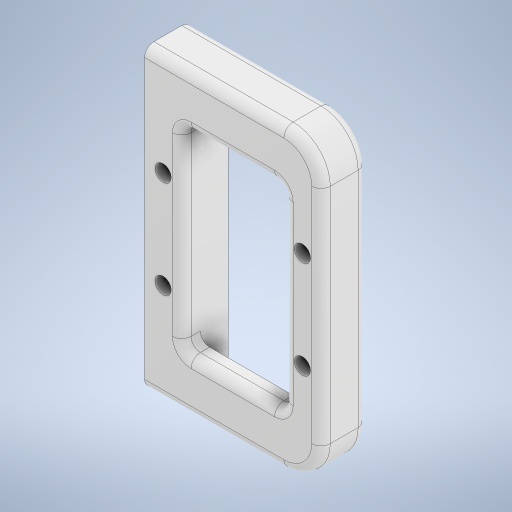
# Autodesk Inventor part: CoxaLeft
Saved by Autodesk Inventor 2024 (Build 280153000, 153)
## iProperties
Created: 2026-01-13
Part Number: CoxaLeft
Material: Generic
Document SubType Name: Modeling
Designer: Liam
Density: 1 g/cm^3
Appearance: Default
Author: Liam
Autodesk Inventor part; units mm, degrees
ref_plane "YZ Plane" through (0, 0, 0) normal (1, 0, 0) x (0, 1, 0)
ref_plane "XZ Plane" through (0, 0, 0) normal (0, 1, 0) x (-1, 0, 0)
ref_plane "XY Plane" through (0, 0, 0) normal (0, 0, 1) x (1, 0, 0)
sketch "Sketch1" plane through (0, 0, 0) normal (0, 0, 1) x (1, 0, 0)
  line L0 (0, 0) -> (22, 0)
  line L1 (22, 0) -> (22, 42)
  line L2 (22, 42) -> (0, 42)
  line L3 (0, 42) -> (0, 0)
  line L4 (-8, 50) -> (30, 50)
  line L5 (30, 50) -> (30, -8)
  line L6 (30, -8) -> (-8, -8)
  line L7 (-8, -8) -> (-8, 50)
  line L8 (0, 21) -> (22, 21) construction
  line L9 (11, 0) -> (11, 42) construction
  circle A0 centre (26, 10.5) radius 1.75
  circle A1 centre (26, 31.5) radius 1.75
  circle A2 centre (-4, 10.5) radius 1.75
  circle A3 centre (-4, 31.5) radius 1.75
  line L10 (0, 50) -> (22, 50)
  line L11 (22, 42) -> (0, 42)
  line L12 (0, 0) -> (22, 0)
  line L13 (22, -8) -> (0, -8)
  line L14 (5.4779, 42) -> (18.0265, 42)
  line L15 (5.4779, 0) -> (19.7232, 0)
  line L16 (0, 42) -> (0, 50)
  line L17 (22, 42) -> (22, 50)
  line L18 (0, 0) -> (0, -8)
  line L19 (22, 0) -> (22, -8)
  line L20 (-8, 50) -> (30, 50)
  line L21 (30, 50) -> (30, 53)
  line L22 (30, 53) -> (-8, 53)
  line L23 (-8, 53) -> (-8, 50)
  line L24 (-8, -8) -> (30, -8)
  line L25 (30, -8) -> (30, -11)
  line L26 (30, -11) -> (-8, -11)
  line L27 (-8, -11) -> (-8, -8)
  dimension "d0" = 42
  dimension "d2" = 8
  dimension "d3" = 3.5
  dimension "d4" = 10.5
  dimension "d5" = 4
  dimension "d6" = 8
  dimension "d15" = 22
  dimension "d16" = 22
  dimension "d17" = 22
  dimension "d18" = 3
  dimension "d19" = 38
  dimension "d20" = 38
  dimension "d21" = 3
  constraints: 56 end point, 11 parallel, 7 horizontal, 6 perpendicular, 4 centre point, 4 midpoint, 4 point on line, 3 symmetric about line, 1 vertical, 6 other
  measures "d0" distance of L0.end L1.end
  measures "d2" distance between parallel lines of L4 L2
  measures "d3" diameter of A0
  measures "d4" distance from line of A0.centre L8
  measures "d5" distance from line of L1 A0.centre
  measures "d6" distance of L11.end L10.start
  measures "d15" distance of L1.end L2.end
  measures "d16" distance between parallel lines of L17 L16
  measures "d17" distance between parallel lines of L19 L18
  measures "d18" distance between parallel lines of L22 L4
  measures "d19" distance between parallel lines of L23 L21
  measures "d20" distance of L25.end L26.end
  measures "d21" distance of L24.end L25.end
extrude "Extrusion1" add sketch "Sketch1" along normal blind 10 contours L18 L6 L7 L4 L16 L3 | L0 L19 L6 L18 | L16 L4 L17 L2 | L6 L25 L26 L27 | L4 L23 L22 L21 | L19 L1 L17 L4 L5 L6
extrude "Extrusion2" cut sketch "Sketch1" along normal blind 6 contours L0 L19 L6 L18 | L16 L4 L17 L2
fillet "Fillet1" radius 8 2 edges at (30, -11, 5) (30, 53, 5)
fillet "Fillet2" radius 2 4 edges at (0, 42, 8) (0, 0, 8) (22, 0, 8) (22, 42, 8)
fillet "Fillet3" radius 2 12 edges at (27.6569, 50.6569, 10) (27.6569, -8.6569, 10) (7, -11, 10) (7, 53, 10) (27.6569, 50.6569, 0) (27.6569, -8.6569, 0) (7, -11, 0) (7, 53, 0) (11, 0, 10) (0, 21, 10) (11, 42, 10) (22, 21, 10)
equation "\"d0\" = MOUNT_LENGTH"
equation "\"d2\" = MOUNT_THICKNESS"
equation "\"d3\" = ThroughDiameter"
equation "\"d4\" = 0.25 * MOUNT_LENGTH"
equation "\"d5\" = 0.5 * MOUNT_THICKNESS"
equation "\"d15\" = MOUNT_WIDTH"
equation "\"d18\" = -0.5 * MOUNT_LENGTH + 0.5 * COXA_JOINT_LENGTH"
equation "\"d19\" = MOUNT_WIDTH + 2 * MOUNT_THICKNESS"
equation "\"d20\" = MOUNT_WIDTH + 2 * MOUNT_THICKNESS"
equation "\"d21\" = -0.5 * MOUNT_LENGTH + 0.5 * COXA_JOINT_LENGTH"
equation "\"d22\" = OUTER_FILLET"
equation "\"d13\" = INNER_FILLET"
equation "\"d23\" = INNER_FILLET"
equation "\"ThroughDiameter\" = 3.5"
equation "\"MOUNT_LENGTH\" = 42"
equation "\"MOUNT_THICKNESS\" = 8"
equation "\"MOUNT_WIDTH\" = 22"
equation "\"COXA_JOINT_LENGTH\" = 48"
equation "\"OUTER_FILLET\" = 8"
equation "\"INNER_FILLET\" = 2"
body "Solid1"
